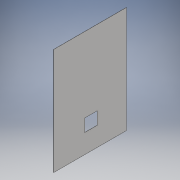
# Autodesk Inventor part: cover 2
Saved by Autodesk Inventor 2018 (Build 220112000, 112)
## iProperties
Created: 2018-03-20
Part Number: cover 2
Material: Generic
Document SubType Name: Modeling
Designer: p446024
Density: 1 g/cm^3
Appearance: Default
Author: p446024
Autodesk Inventor part; units mm, degrees
ref_plane "YZ Plane" through (0, 0, 0) normal (1, 0, 0) x (0, 1, 0)
ref_plane "XZ Plane" through (0, 0, 0) normal (0, 1, 0) x (-1, 0, 0)
ref_plane "XY Plane" through (0, 0, 0) normal (0, 0, 1) x (1, 0, 0)
sketch "Sketch1" plane through (0, 0, 0) normal (0, 0, 1) x (1, 0, 0)
  line L0 (0, 0) -> (1.6, 0)
  line L1 (1.6, 0) -> (1.6, 700)
  line L2 (1.6, 700) -> (0, 700)
  line L3 (0, 700) -> (0, 0)
  dimension "d0" = 700
  dimension "d1" = 1.6
  constraints: 8 end point, 2 parallel, 1 horizontal, 1 perpendicular
  measures "d0" distance of L0.end L1.end
  measures "d1" distance of L1.end L2.end
extrude "Extrusion1" add sketch "Sketch1" along normal blind 1100
sketch "Sketch2" plane through (1.6, 0, 0) normal (0, -1, 0) x (1, 0, 0)
  line L0 (-1.6, 0) -> (-1.6, 1100) projected
  line L1 (-1.6, 0) -> (0, 0) projected
  line L2 (-1.6, 0) -> (0, 0) projected
  line L3 (0, 0) -> (0, 1100) projected
  line L4 (-1.6, 1100) -> (0, 1100) projected
  line L5 (-1.6, 0) -> (-1.6, 1100) projected
extrude "Extrusion2" add sketch "Sketch2" along normal blind 50
sketch "Sketch3" plane through (1.6, 700, 1100) normal (1, 0, 0) x (0, 0, -1)
  line L0 (1100, 0) -> (1100, -750) projected
  line L1 (1100, -427.9985) -> (1362.866, -427.9985) construction
  line L2 (0, -750) -> (1100, -750) projected
  line L3 (772.134, -300.688) -> (772.134, -430.688)
  line L4 (772.134, -430.688) -> (902.134, -430.688)
  line L5 (902.134, -430.688) -> (902.134, -300.688)
  line L6 (772.134, -300.688) -> (902.134, -300.688)
  point P0 (1100, -700)
  dimension "d11" = 130
  dimension "d12" = 130
  dimension "d13" = 130
  constraints: 10 end point, 2 horizontal, 1 perpendicular, 1 point on line
  measures "d11" distance of L3.start L3.end
  measures "d12" distance of L3.end L4.end
  measures "d13" distance of L4.end L5.end
extrude "Extrusion3" cut sketch "Sketch3" against normal through all
body "Solid1"
